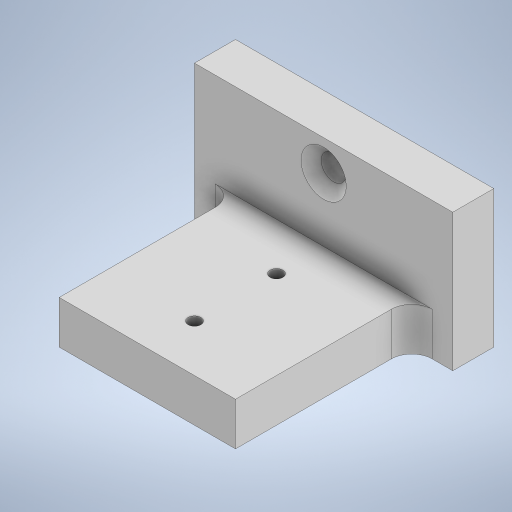
# Autodesk Inventor part: Camera Holder
Saved by Autodesk Inventor 2024 (Build 280153000, 153)
## iProperties
Created: 2026-03-12
Part Number: Camera Holder
Material: Generic
Document SubType Name: Modeling
Designer: Nathan
Density: 1 g/cm^3
Appearance: Default
Author: Nathan
Autodesk Inventor part; units mm, degrees
ref_plane "YZ Plane" through (0, 0, 0) normal (1, 0, 0) x (0, 1, 0)
ref_plane "XZ Plane" through (0, 0, 0) normal (0, 1, 0) x (-1, 0, 0)
ref_plane "XY Plane" through (0, 0, 0) normal (0, 0, 1) x (1, 0, 0)
sketch "Sketch1" plane through (0, 0, 0) normal (0, 1, 0) x (-1, 0, 0)
  line L0 (21.5, 21.5) -> (-21.5, 21.5)
  line L1 (-21.5, 21.5) -> (-21.5, -21.5)
  line L2 (-21.5, -21.5) -> (21.5, -21.5)
  line L3 (21.5, -21.5) -> (21.5, 21.5)
  line L4 (21.5, 21.5) -> (-21.5, -21.5) construction
  line L5 (-21.5, 21.5) -> (21.5, -21.5) construction
  point P0 (0, 0)
  dimension "d0" = 43
  dimension "d1" = 43
  constraints: 12 end point, 2 midpoint, 2 parallel, 1 horizontal, 1 perpendicular
  measures "d0" distance of L2.end L1.end
  measures "d1" distance of L1.end L0.end
extrude "Extrusion1" add sketch "Sketch1" along normal blind 10
sketch "Sketch3" plane through (0, 0, 0) normal (0, 1, 0) x (-1, 0, 0)
  line L0 (31.5, -31.5) -> (-31.5, -31.5)
  line L1 (-31.5, -31.5) -> (-31.5, 31.5)
  line L2 (-31.5, 31.5) -> (31.5, 31.5)
  line L3 (31.5, 31.5) -> (31.5, -31.5)
  line L4 (31.5, -31.5) -> (-31.5, 31.5) construction
  line L5 (-31.5, -31.5) -> (31.5, 31.5) construction
  line L6 (-21.5, 21.5) -> (-21.5, -21.5) projected
  line L7 (21.5, 21.5) -> (-21.5, 21.5)
  line L8 (-21.5, 21.5) -> (-21.5, -21.5)
  line L9 (-21.5, -21.5) -> (21.5, -21.5)
  line L10 (21.5, -21.5) -> (21.5, 21.5)
  line L11 (21.5, 21.5) -> (-21.5, -21.5) construction
  line L12 (-21.5, 21.5) -> (21.5, -21.5) construction
  point P0 (0, 0)
  dimension "d13" = 63
  dimension "d14" = 63
  constraints: 24 end point, 4 midpoint, 4 parallel, 2 horizontal, 2 perpendicular
  measures "d13" distance of L1.end L2.end
  measures "d14" distance of L0.end L1.end
extrude "Extrusion2" add sketch "Sketch3" along normal blind 15
sketch "Sketch4" plane through (0, 15, 0) normal (0, 1, 0) x (1, 0, 0)
  line L0 (31.5, -31.5) -> (31.5, 31.5) projected
  line L1 (-31.5, 31.5) -> (31.5, 31.5)
  line L2 (31.5, 31.5) -> (31.5, 21.5)
  line L3 (31.5, 21.5) -> (-31.5, 21.5)
  line L4 (-31.5, 21.5) -> (-31.5, 31.5)
  point P0 (0, 0)
  dimension "d17" = 10
  constraints: 8 end point, 2 parallel, 1 horizontal, 1 perpendicular, 1 point on line
  measures "d17" distance of L1.end L2.end
extrude "Extrusion3" add sketch "Sketch4" along normal blind 18
sketch "Sketch5" plane through (31.5, 0, -31.5) normal (0, 0, -1) x (-1, 0, 0)
  line L0 (0, 15) -> (0, 33) construction
  line L1 (63, 15) -> (63, 33) construction
  line L2 (0, 33) -> (63, 33) construction
  line L3 (63, 33) -> (63, 18) construction
  line L4 (63, 18) -> (0, 18) construction
  line L5 (0, 18) -> (0, 33) construction
  line L6 (0, 18) -> (0, 25.5) construction
  line L7 (0, 29.25) -> (63, 29.25)
  line L8 (63, 29.25) -> (63, 21.75)
  line L9 (63, 21.75) -> (0, 21.75)
  line L10 (-63, 29.25) -> (63, 21.75) construction
  line L11 (63, 29.25) -> (-63, 21.75) construction
  line L12 (0, 29.25) -> (0, 21.75)
  line L13 (31.5, 33) -> (31.5, 25.5) construction
  line L14 (31.5, 25.5) -> (11.5, 25.5) construction
  line L15 (31.5, 25.5) -> (51.5, 25.5) construction
  circle A0 centre (11.5, 25.5) radius 2.5
  circle A1 centre (51.5, 25.5) radius 2.5
  point P0 (31.5, 0)
  dimension "d20" = 15
  dimension "d21" = 7.5
  dimension "d22" = 7.5
  dimension "d33" = 20
  dimension "d34" = 20
  dimension "d35" = 5
  dimension "d36" = 5
  constraints: 28 end point, 4 horizontal, 4 midpoint, 3 parallel, 2 centre point, 2 coincident, 2 perpendicular, 2 point on line, 1 vertical
  measures "d20" distance of L2.end L3.end
  measures "d21" distance of L4.end L6.end
  measures "d22" distance of L7.end L8.end
  measures "d33" distance of L13.end L14.end
  measures "d34" distance of L13.end L15.end
  measures "d35" diameter of A0
  measures "d36" diameter of A1
sketch "Sketch6" plane through (-21.5, 10, -21.5) normal (0, 0, 1) x (1, 0, 0)
  line L0 (-10, 23) -> (53, 23) construction
  line L1 (53, 23) -> (53, 15.5) construction
  line L2 (53, -10) -> (53, 23) construction
  line L3 (53, 15.5) -> (-10, 15.5) construction
  line L4 (-10, -10) -> (-10, 23) construction
  line L5 (21.5, 23) -> (21.5, 15.5) construction
  point P0 (21.5, -10)
  dimension "d25" = 7.5
  constraints: 6 end point, 2 midpoint, 2 point on line, 1 perpendicular
  measures "d25" distance of L0.end L1.end
hole "Hole2" at (0, 25.5, -21.5) direction (0, 0, -1) diameter 6.1 end through all countersink diameter 11 countersink angle 90 clearance for "Countersunk Flat Head Screw ISO 2009/7046" size "M6" standard "ISO"
extrude "Extrusion5" cut sketch "Sketch5" against normal blind 6 contours A0 | A1
sketch "Sketch7" plane through (0, 15, 0) normal (0, 1, 0) x (1, 0, 0)
  line L0 (-31.5, -31.5) -> (31.5, -31.5) projected
  line L1 (21.5, 21.5) -> (-21.5, 21.5) projected
  line L2 (-31.5, -31.5) -> (-21.5, -31.5)
  line L3 (-21.5, -31.5) -> (-21.5, 21.5)
  line L4 (-21.5, 21.5) -> (-31.5, 21.5)
  line L5 (-31.5, 21.5) -> (-31.5, -31.5)
  point P0 (0, 0)
  constraints: 8 end point, 2 parallel, 1 horizontal, 1 perpendicular
extrude "Extrusion6" add sketch "Sketch7" along normal up to surface (18 mm away)
fillet "Fillet1" radius 18 1 edges at (-26.5, 33, 31.5)
sketch "Sketch9" plane through (0, 33, 0) normal (0, 1, 0) x (1, 0, 0)
  line L0 (21.5, 21.5) -> (-21.5, 21.5) construction
  line L1 (-21.5, 21.5) -> (-31.5, 21.5) construction
  line L2 (-31.5, 31.5) -> (-31.5, -13.5) construction
  line L3 (31.5, -31.5) -> (31.5, 21.5) projected
  line L4 (-31.5, 21.5) -> (31.5, 21.5)
  line L5 (31.5, 21.5) -> (31.5, -31.5)
  line L6 (31.5, -31.5) -> (-31.5, -31.5)
  line L7 (-31.5, -31.5) -> (-31.5, 21.5)
  point P0 (0, 0)
  constraints: 10 end point, 2 horizontal, 2 parallel, 1 perpendicular, 1 point on line
extrude "Extrusion7" cut sketch "Sketch9" against normal up to surface (23 mm away)
sketch "Sketch10" plane through (0, 10, 0) normal (0, 1, 0) x (1, 0, 0)
  line L0 (21.5, -21.5) -> (-21.5, -21.5)
  line L1 (-21.5, -21.5) -> (-21.5, 21.5)
  line L2 (-21.5, 21.5) -> (21.5, 21.5)
  line L3 (21.5, 21.5) -> (21.5, -21.5)
  line L4 (21.5, -21.5) -> (-21.5, 21.5) construction
  line L5 (-21.5, -21.5) -> (21.5, 21.5) construction
  line L6 (31.5, -31.5) -> (-31.5, -31.5) projected
  line L7 (-31.5, 31.5) -> (31.5, 31.5)
  line L8 (31.5, 31.5) -> (31.5, -31.5)
  line L9 (31.5, -31.5) -> (-31.5, -31.5)
  line L10 (-31.5, -31.5) -> (-31.5, 31.5)
  line L11 (-31.5, 31.5) -> (31.5, -31.5) construction
  line L12 (31.5, 31.5) -> (-31.5, -31.5) construction
  line L13 (-31.5, 21.5) -> (31.5, 21.5) projected
  line L14 (21.5, 21.5) -> (31.5, 21.5)
  line L15 (-31.5, 21.5) -> (-21.5, 21.5)
  point P0 (0, 0)
  dimension "d55" = 43
  dimension "d56" = 43
  constraints: 28 end point, 4 midpoint, 4 parallel, 2 horizontal, 2 perpendicular
  measures "d55" distance of L1.end L2.end
  measures "d56" distance of L0.end L1.end
extrude "Extrusion8" cut sketch "Sketch10" against normal through all contours L3 L13 L8 L6 L10 L1 L0
fillet "Fillet2" radius 5 2 edges at (21.5, 5, -21.5) (-21.5, 5, -21.5)
sketch "Sketch11" plane through (0, 0, 0) normal (0, -1, 0) x (1, 0, 0)
  line L0 (21.5, 21.5) -> (-21.5, 21.5) projected
  line L1 (17, -31.5) -> (23, -31.5) projected
  line L2 (-21.5, 21.5) -> (21.5, 21.5)
  line L3 (21.5, 21.5) -> (21.5, -16.5)
  line L4 (21.5, -31.5) -> (-21.5, -31.5)
  line L5 (-21.5, -16.5) -> (-21.5, 21.5)
  line L6 (31.5, -21.5) -> (31.5, -31.5) projected
  line L7 (-26.5, -21.5) -> (-31.5, -21.5)
  line L8 (-31.5, -21.5) -> (-31.5, -31.5)
  line L9 (-31.5, -31.5) -> (31.5, -31.5)
  line L10 (31.5, -31.5) -> (31.5, -21.5)
  arc A0 (-26.5, -21.5) -> (-21.5, -16.5) centre (-26.5, -16.5) ccw
  arc A1 (21.5, -16.5) -> (26.5, -21.5) centre (26.5, -16.5) ccw projected
  arc A2 (21.5, -16.5) -> (26.5, -21.5) centre (26.5, -16.5) ccw
  line L11 (26.5, -21.5) -> (31.5, -21.5)
  point P0 (0, 0)
  dimension "d64" = 63
  dimension "d65" = 5
  constraints: 18 end point, 5 point on circle, 5 point on line, 4 parallel, 4 tangent, 3 horizontal, 2 centre point, 2 perpendicular, 1 coincident
  measures "d64" distance of L9.end L8.end
  measures "d65" radius of A0
extrude "Extrusion9" add sketch "Sketch11" along normal blind 0.5
sketch "Sketch12" plane through (0, -0.5, 0) normal (0, -1, 0) x (1, 0, 0)
  line L0 (0, 0) -> (0, 10)
  line L1 (0, 0) -> (0, -10)
  dimension "d68" = 10
  dimension "d69" = 10
  constraints: 4 end point, 2 vertical
  measures "d68" distance of L0.start L0.end
  measures "d69" distance of L0.start L1.end
hole "Hole4" at (0, -0.5, -10) at (0, -0.5, 10) direction (0, 1, 0) diameter 3.1 end through all countersink diameter 5.8 countersink angle 90 clearance for "Countersunk Flat Head Screw ISO 2009/7046" size "M3" standard "ISO"
body "Solid1"
